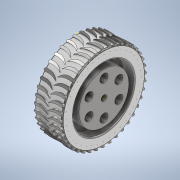
# Autodesk Inventor part: wheel
Saved by Autodesk Inventor 2021 (Build 250183000, 183)
## iProperties
Created: 2021-07-14
Part Number: wheel
Material: Steel, Mild
Document SubType Name: Modeling
Designer: HP
Density: 7.85 g/cm^3
Appearance: Semi-Polished
Author: HP
Autodesk Inventor part; units mm, degrees
ref_plane "YZ Plane" through (0, 0, 0) normal (1, 0, 0) x (0, 1, 0)
ref_plane "XY Plane" through (0, 0, 0) normal (0, 0, 1) x (1, 0, 0)
sketch "Sketch1" plane through (0, 0, 0) normal (1, 0, 0) x (0, 1, 0)
  circle A0 centre (0, 0) radius 75
  dimension "d0" = 150
  constraints: 1 centre point, 1 coincident
  measures "d0" diameter of A0
extrude "Extrusion1" add sketch "Sketch1" along normal blind 50
fillet "Fillet1" radius 2 2 edges at (50, -75, 0) (0, -75, 0)
sketch "Sketch2" plane through (50, 0, 0) normal (1, 0, 0) x (0, 0, -1)
  circle A0 centre (0, 0) radius 55
  circle A1 centre (0, 0) radius 45
  dimension "d4" = 110
  dimension "d5" = 90
  constraints: 2 centre point, 2 coincident
  measures "d4" diameter of A0
  measures "d5" diameter of A1
extrude "Extrusion2" cut sketch "Sketch2" against normal blind 20
sketch "Sketch3" plane through (0, 0, 0) normal (-1, 0, 0) x (0, 0, 1)
  circle A0 centre (0, 0) radius 55
  circle A1 centre (0, 0) radius 47.5
  dimension "d8" = 110
  dimension "d9" = 95
  constraints: 2 centre point, 2 coincident
  measures "d8" diameter of A0
  measures "d9" diameter of A1
extrude "Extrusion3" cut sketch "Sketch3" against normal blind 20
sketch "Sketch6" plane through (20, 0, 0) normal (-1, 0, 0) x (0, 0, 1)
  circle A0 centre (0, 31.1021) radius 7.5
  circle A1 centre (-26.9352, 15.551) radius 7.5
  circle A2 centre (-26.9352, -15.551) radius 7.5
  circle A3 centre (0, -31.1021) radius 7.5
  circle A4 centre (26.9352, -15.551) radius 7.5
  circle A5 centre (26.9352, 15.551) radius 7.5
  point P0 (0, 0)
  point P1 (0, 0)
  point P2 (0, 0)
  point P3 (0, 0)
  point P4 (0, 0)
  point P5 (0, 0)
  dimension "d18" = 15
  dimension "d21" = 360
  constraints: 6 centre point, 2 coincident, 17 other
  measures "d18" diameter of A0
extrude "Extrusion6" cut sketch "Sketch6" against normal mid plane 100
sketch "Sketch7" plane through (50, 0, 0) normal (1, 0, 0) x (0, 0, -1)
  circle A0 centre (0, 0) radius 5
  dimension "d25" = 10
  constraints: 1 centre point, 1 coincident
  measures "d25" diameter of A0
extrude "Extrusion7" cut sketch "Sketch7" along normal mid plane 100
fillet "Fillet2" radius 2 2 edges at (0, 0, -55) (50, 0, 55)
sketch "Sketch8" plane through (0, 0, 0) normal (0, 1, 0) x (-1, 0, 0)
  point P0 (0, 0)
sketch "Sketch9" plane through (50, 0, 0) normal (1, 0, 0) x (0, 0, -1)
  point P0 (0, 0)
ref_plane "Work Plane2" through (0, 76.5, 0) normal (0, 1, 0) x (-1, 0, 0)
sketch "Sketch10" plane through (0, 76.5, 0) normal (0, 1, 0) x (-1, 0, 0)
  point P0 (0, 0)
sketch "Sketch11" plane through (0, 76.5, 0) normal (0, 1, 0) x (-1, 0, 0)
  arc A0 (-25, 0) -> (-1.9507, -3.8182) centre (-7.8203, 32.229) ccw
  arc A1 (-25, 0) -> (-2.03, -8.2582) centre (-7.8334, 11.6741) ccw
  arc A2 (-47.9934, -9.1083) -> (-24.8902, -5.5411) centre (-41.566, 25.8627) ccw
  arc A3 (-46.6843, -13.9675) -> (-24.8902, -5.5411) centre (-41.7717, 5.724) ccw
  arc A4 (-3.4779, -8.6238) -> (-2.9398, -3.9654) centre (-2.8847, -6.332) ccw
  line L0 (0, -47.5) -> (0, 47.5) projected
  arc A5 (-47.9934, -9.1083) -> (-46.6843, -13.9675) centre (-47.3388, -11.5379) ccw
  point P0 (0, 0)
  constraints: 14 point on circle, 6 centre point
extrude "Extrusion8" add sketch "Sketch11" against normal blind 10 separate body contours A2 A3 A5
extrude "Extrusion9" add sketch "Sketch11" against normal blind 10 separate body contours A0 A4 A1
fillet "Fillet3" radius 0.2 2 edges at (24.8902, 71.5, -5.5411) (25, 71.5, 0)
fillet "Fillet4" radius 0.2 6 edges at (25.3633, 76.5, -5.96) (36.5385, 76.5, -9.3368) (34.8328, 76.5, -13.348) (24.5119, 76.5, -0.4289) (13.8759, 76.5, -3.7874) (15.1684, 76.5, -7.7469)
pattern_circular "Circular Pattern1" count 40 over 360 about axis through (0, 0, 0) along (1, 0, 0) of "Extrusion9", "Extrusion8" bodies 3
body "Solid1"
body "Solid2"
body "Solid3"
